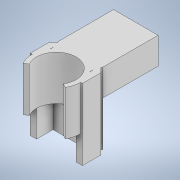
# Autodesk Inventor part: motor holder v2
Saved by Autodesk Inventor 2022 (Build 260153000, 153)
## iProperties
Created: 2021-11-11
Part Number: motor holder v2
Material: Generic
Document SubType Name: Modeling
Designer: a-dubs
Density: 1 g/cm^3
Appearance: Default
Author: a-dubs
Autodesk Inventor part; units mm, degrees
ref_plane "YZ Plane" through (0, 0, 0) normal (1, 0, 0) x (0, 1, 0)
ref_plane "XZ Plane" through (0, 0, 0) normal (0, 1, 0) x (-1, 0, 0)
ref_plane "XY Plane" through (0, 0, 0) normal (0, 0, 1) x (1, 0, 0)
sketch "Sketch1" plane through (0, 0, 0) normal (0, 1, 0) x (-1, 0, 0)
  line L0 (0, 0) -> (15, 0)
  line L1 (15, 0) -> (15, 34)
  line L2 (15, 34) -> (0, 34)
  line L3 (0, 34) -> (0, 0)
  line L4 (7.5, 34) -> (7.5, 36.5)
  line L5 (7.5, 36.5) -> (7.5, 47.61)
  circle A0 centre (7.5, 47.61) radius 11.11
  circle A1 centre (7.5, 47.61) radius 13.61
  line L6 (7.5, 47.61) -> (19.2866, 54.415)
  line L7 (7.5, 47.61) -> (21.11, 47.61) construction
  line L8 (7.5, 47.61) -> (-4.2866, 54.415)
  line L9 (7.5, 47.61) -> (21.11, 47.61) construction
  line L10 (15, 34) -> (18.5355, 37.5355)
  line L11 (15, 34) -> (20, 34) construction
  line L12 (18.5355, 37.5355) -> (18.5355, 39.6445)
  line L13 (0, 34) -> (-3.5355, 37.5355)
  line L14 (-3.5355, 37.5355) -> (-3.5355, 39.6445)
  line L15 (7.5, 47.61) -> (7.5, 56.86)
  line L16 (7.5, 56.86) -> (17.4835, 56.86)
  line L17 (7.5, 56.86) -> (-2.4835, 56.86)
  line L18 (7.5, 47.61) -> (-6.11, 47.61)
  line L19 (7.5, 47.61) -> (7.5, 38.36)
  line L20 (7.5, 38.36) -> (17.4835, 38.36)
  line L21 (7.5, 38.36) -> (-2.4835, 38.36)
  line L22 (7.5, 38.36) -> (-3.61, 38.36)
  line L23 (-3.61, 38.36) -> (-3.61, 47.61)
  line L24 (-3.61, 47.61) -> (-3.61, 56.86)
  line L25 (-3.61, 56.86) -> (-2.4835, 56.86)
  line L26 (7.5, 56.86) -> (18.61, 56.86)
  line L27 (18.61, 56.86) -> (18.61, 47.61)
  line L28 (7.5, 38.36) -> (18.61, 38.36)
  line L29 (18.61, 38.36) -> (18.61, 47.61)
  line L30 (7.5, 0) -> (7.5, 3)
  line L31 (7.5, 3) -> (0, 3)
  line L32 (7.5, 3) -> (15, 3)
  line L33 (7.5, 3) -> (20, 3)
  line L34 (7.5, 3) -> (-5, 3)
  line L35 (7.5, 34) -> (20, 34)
  line L36 (7.5, 34) -> (-5, 34)
  line L37 (-5, 34) -> (-5, 3)
  line L38 (20, 3) -> (20, 34)
  line L39 (18.61, 38.36) -> (22.1455, 34.8245)
  line L40 (-3.61, 56.86) -> (-7.1455, 60.3955)
  line L41 (22.1455, 34.8245) -> (-7.1455, 34.8245)
  line L42 (-7.1455, 34.8245) -> (-7.1455, 60.3955)
  line L43 (-7.1455, 60.3955) -> (22.1455, 60.3955)
  line L44 (22.1455, 60.3955) -> (22.1455, 34.8245)
  line L45 (-3.5355, 37.5355) -> (-5, 34)
  line L46 (18.5355, 37.5355) -> (20, 34)
  line L47 (7.5, 47.61) -> (-7.1455, 47.61)
  line L48 (7.5, 47.61) -> (22.1455, 47.61)
  point P0 (17.1215, 53.165)
  point P1 (-2.1215, 53.165)
  point P2 (0, 34)
  point P3 (0, 3)
  point P4 (0, 34)
  point P5 (2.835, 60.3955)
  point P6 (-4.6585, 34.8245)
  point P7 (-3.5355, 38.36)
  point P8 (-3.61, 39.7487)
  point P9 (-3.61, 55.4713)
  point P10 (12.165, 60.3955)
  point P11 (18.61, 55.4713)
  point P12 (18.61, 39.7487)
  point P13 (18.5355, 38.36)
  point P14 (19.6585, 34.8245)
  point P15 (18.61, 47.61)
  dimension "d0" = 15
  dimension "d1" = 34
  dimension "d2" = 2.5
  dimension "d3" = 11.11
  dimension "d4" = 30
  dimension "d5" = 150
  dimension "d6" = 5
  dimension "d7" = 45
  dimension "d10" = 9.25
  dimension "d11" = 11.11
  dimension "d12" = 11.11
  dimension "d13" = 11.11
  dimension "d14" = 3
  dimension "d15" = 12.5
  dimension "d16" = 5
  dimension "d17" = 5
  constraints: 98 end point, 13 point on line, 9 horizontal, 8 perpendicular, 5 symmetric about line, 4 equal length, 4 midpoint, 3 parallel, 3 point on circle, 3 vertical, 2 coincident, 1 centre point, 1 collinear, 1 tangent, 9 other
  measures "d0" distance of L0.start L0.end
  measures "d1" distance of L0.end L1.end
  measures "d2" distance of L4.start L4.end
  measures "d3" distance of L4.end L5.end
  measures "d4" angle of L7 L6
  measures "d5" angle of L9 L8
  measures "d6" distance of L1.end L10.end
  measures "d7" angle of L11 L10
  measures "d10" distance of L6.start L15.end
  measures "d11" distance of L19.end L22.end
  measures "d12" distance of L15.end L26.end
  measures "d13" distance of L19.end L28.end
  measures "d14" distance of L30.start L30.end
  measures "d15" distance of L30.end L33.end
  measures "d16" distance of L28.end L39.end
  measures "d17" distance of L24.end L40.end
extrude "Extrusion1" add sketch "Sketch1" along normal blind 15 and the other way blind 10 contours L13 L41 A1 L2 | L36 L45 L41 L13 | A1 L41 L10 L2 | A1 L41 L4 | L4 L41 A1 | L41 L45 L13 | L13 L14 L22 A1 L41 | L10 L41 L46 L35 | L41 A1 L21 A0 L4 | L4 A0 L20 A1 L41 | A1 L28 L12 L10 L41 | L45 L41 L42 L47 A1 L23 L22 L14 | L10 L46 L41 | L22 L14 A1 | A1 L23 A0 L21 | L20 A0 L29 A1 | A1 L12 L28 | L12 L28 L39 L41 L46 | L39 L29 A1 L48 L44 | L24 L8 A0 | L23 A1 L18 | L18 A1 L8 L24 | A0 L6 L27 | L48 A1 L29 | L27 L6 A1 L48
extrude "Extrusion2" add sketch "Sketch1" along normal blind 15 contours L34 L37 L36 L3 | L3 L2 L1 L32 L31 | L1 L35 L38 L33
extrude "Extrusion3" add sketch "Sketch1" against normal blind 15 from surface at -10 contours L13 L41 A1 L2 | L36 L45 L41 L13 | A1 L41 L10 L2 | A1 L41 L4 | L4 L41 A1 | L41 L45 L13 | L13 L14 L22 A1 L41 | L10 L41 L46 L35 | L41 A1 L21 A0 L4 | L4 A0 L20 A1 L41 | A1 L28 L12 L10 L41 | L45 L41 L42 L47 A1 L23 L22 L14 | L10 L46 L41 | A0 L21 L5 | L5 L20 A0 | L12 L28 L39 L41 L46 | L39 L29 A1 L48 L44 | L23 A1 L18 | L48 A1 L29
chamfer "Chamfer2" distance 2.4 angle 45 2 edges at (7.1455, -5, 34.8245) (-22.1455, -5, 34.8245)
body "Solid1"
